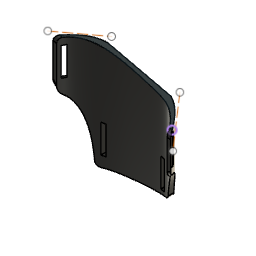
Back Hand Exo Bottom v4-flex material version v2 (Autodesk Fusion 360 design; units mm, degrees)
Autodesk Fusion 360 part; units mm, degrees
sketch "Base" plane through (0, 0, 0) normal (0, 0, 1) x (1, 0, 0)
  spline S0 degree 5 poles (14.4752, -0.0001) (14.6938, 0.8156) (15.231, 2.4269) (16.338, 4.7834) (18.4093, 7.7764) (22.0639, 11.0963) (26.9085, 13.7883) (33.3851, 15.6119) (41.8139, 16.4597) (51.3186, 16.5539) (60.7436, 16.1818) (68.8276, 15.6297) (74.9011, 14.9312) (78.8611, 13.937) (82.7401, 11.6359) (87.0744, 7.9841) (90.1424, 4.6022) (91.6876, 2.194) (92.2847, 0.711) (92.4752, 0) knots 0 0 0 0 0 0 0.066667 0.133333 0.2 0.266667 0.333333 0.4 0.466667 0.533333 0.6 0.666667 0.733333 0.8 0.866667 0.933333 1 1 1 1 1 1
  line L0 (12.4519, -7.5513) -> (16.4985, 7.551)
  line L1 (0, 0) -> (130, 0) construction
  line L2 (90.742, 6.4684) -> (94.2084, -6.4684)
  line L3 (72.0197, 16) -> (83.6365, 12)
  line L4 (20.0406, 11.0956) -> (36.9098, 16.9041)
  line L5 (28.4752, 32.4834) -> (28.4752, -47.2676) construction
  line L6 (79.3904, 33.3073) -> (79.3904, -47.7619) construction
  line L7 (14.4752, -0.0001) -> (11.9752, 0)
  line L8 (94.9752, 0) -> (92.4752, 0)
  line L9 (30.9752, 19.2841) -> (75.9752, 19.2841)
  line L10 (53.4752, 19.2841) -> (53.4752, -22.3142) construction
  spline S1 degree 5 poles (11.9752, 0) (12.2539, 0.5131) (12.8175, 1.532) (13.6807, 3.039) (14.8682, 5.0045) (16.4196, 7.3808) (18.0501, 9.6607) (19.7785, 11.8195) (21.6298, 13.823) (23.6348, 15.6281) (25.8277, 17.186) (27.7599, 18.1954) (29.322, 18.8009) (30.4155, 19.1347) (30.9752, 19.2841) knots 0 0 0 0 0 0 0.1 0.2 0.3 0.4 0.5 0.6 0.7 0.8 0.9 1 1 1 1 1 1
  spline S2 degree 5 poles (75.9752, 19.2841) (76.4009, 19.11) (77.2437, 18.7386) (78.4821, 18.1116) (80.0848, 17.1367) (82.0223, 15.6904) (83.9126, 14.0207) (85.7738, 12.1331) (87.6197, 10.0413) (89.4589, 7.7667) (91.2965, 5.3302) (92.7672, 3.2651) (93.871, 1.6557) (94.6071, 0.5563) (94.9752, 0) knots 0 0 0 0 0 0 0.1 0.2 0.3 0.4 0.5 0.6 0.7 0.8 0.9 1 1 1 1 1 1
  line L11 (27.5864, 18.3796) -> (34.364, 20.1885)
  line L12 (72.8438, 20.5644) -> (79.1066, 18.0038)
  point P0 (28.4752, 13.9999)
  point P1 (77.8281, 14)
  point P2 (20, 12)
  point P3 (84.8904, 13)
  dimension "d1" = 78
  dimension "d3" = 14
  dimension "d4" = 14
  dimension "d5" = 14
  dimension "d6" = 75
  dimension "d7" = 75
  dimension "d8" = 19
  dimension "d9" = 19
  dimension "d10" = 2.5
  dimension "d11" = 2.5
  dimension "d71" = 45
  dimension "d72" = 39
  dimension "d109" = 5.5
  constraint midpoint S0.start L0
  constraint coincident L1.start origin
  constraint horizontal L1
  constraint midpoint S0.end L2
  constraint midpoint P1 L3
  constraint midpoint P0 L4
  constraint coincident L1 L7.end
  constraint coincident L1 L8.start
  constraint perpendicular L1 L5
  constraint vertical L6
  constraint coincident P0 L5
  constraint coincident S0.end L1
  constraint perpendicular L5 L9
  constraint vertical L10
  constraint midpoint L9 L10.start
  constraint midpoint L9.start L11
  constraint midpoint L9.end L12
  measures "d1" distance of S0.start S0.end
  measures "d3" distance of S0.start P0
  measures "d4" distance of S0.start P0
  measures "d5" distance of P1 S0.end
  measures "d6" angle of L0 L1
  measures "d7" angle of L1 L2
  measures "d8" angle of L1 L3
  measures "d9" angle of L1 L4
  measures "d10" distance of S0.end L8.start
  measures "d11" distance of S0.start L7.end
  measures "d71" distance of L9.start L9.end
  measures "d72" distance of S0.start L10
  measures "d109" distance of L6 P3
extrude "Extrude1" add sketch "Base" along normal blind 80
ref_plane "WorkPlane1" through (0, 34, 0) normal (0, 1, 0) x (0, 0, 1)
ref_plane "WorkPlane2" through (0, -2, 0) normal (0, 1, 0) x (0, 0, 1)
sketch "Bottom cut" plane through (0, -2, 0) normal (0, 1, 0) x (1, 0, 0)
  line L0 (104.8084, -92.0022) -> (104.8084, 18.1008) construction
  line L1 (124.2592, 0) -> (-25.481, 0) construction
  line L2 (7.8084, -95.0569) -> (7.8084, 27.3148) construction
  line L3 (10.7244, 0) -> (10.7244, -80) construction
  line L4 (100.7244, 0) -> (100.7244, -80) construction
  line L5 (-40, -55.0042) -> (-40, 40)
  line L6 (-40, 40) -> (120.0224, 40)
  line L7 (120.0224, 40) -> (120.0224, -37.9442)
  line L8 (120.0224, -37.9442) -> (104.8084, -36.9507)
  spline S0 degree 5 poles (4.5707, -55.0042) (5.4547, -54.2774) (7.185, -52.7903) (9.6672, -50.4587) (12.7463, -47.1447) (16.1864, -42.6382) (19.185, -37.7387) (21.7128, -32.42) (23.7655, -26.6781) (25.3732, -20.5401) (26.5747, -14.0405) (27.2401, -8.5774) (27.5837, -4.3416) (27.7449, -1.4573) (27.8084, 0) knots 0 0 0 0 0 0 0.1 0.2 0.3 0.4 0.5 0.6 0.7 0.8 0.9 1 1 1 1 1 1
  spline S1 degree 5 poles (104.8084, -36.9507) (103.912, -36.7934) (102.1545, -36.4375) (99.6247, -35.7798) (96.4678, -34.651) (92.9056, -32.7929) (89.7589, -30.451) (87.057, -27.591) (84.8075, -24.2043) (82.9839, -20.3215) (81.5503, -15.9845) (80.6881, -12.1834) (80.191, -9.1584) (79.9251, -7.0655) (79.8084, -6) knots 0 0 0 0 0 0 0.1 0.2 0.3 0.4 0.5 0.6 0.7 0.8 0.9 1 1 1 1 1 1
  line L9 (79.8084, -6) -> (27.8084, 0)
  line L10 (4.5707, -55.0042) -> (-40, -55.0042)
  point P0 (20.8084, -34.1255)
  point P1 (87.8084, -28.2303)
  dimension "d50" = 20
  dimension "d51" = 13
  dimension "d52" = 17
  dimension "d53" = 25
  dimension "d54" = 97
  dimension "d55" = 6
  constraint vertical L0
  constraint perpendicular L0 L1
  constraint perpendicular L1 L2
  constraint coincident origin L1
  constraint coincident L0 L8.end
  constraint perpendicular L5 L6
  constraint perpendicular L6 L7
  constraint vertical L5
  constraint perpendicular L5 L10
  constraint coincident L1 S0.end
  constraint midpoint L0 L8.end
  measures "d50" distance of L2 S0.end
  measures "d51" distance of L2 P0
  measures "d52" distance of L0 P1
  measures "d53" distance of L0 S1.end
  measures "d54" distance of L0 L2
  measures "d55" distance of L1 S1.end
sketch "Top cut" plane through (0, -2, 0) normal (0, 1, 0) x (1, 0, 0)
  line L0 (101.7244, -58) -> (2.8084, -81)
  line L1 (2.8084, -81) -> (2.8084, -105)
  line L2 (2.8084, -105) -> (101.7244, -105)
  line L3 (101.7244, -105) -> (101.7244, -58)
  line L4 (100.7244, -80) -> (10.7244, -80)
  line L5 (7.8084, -95.0569) -> (7.8084, 27.3148)
  line L6 (100.7244, 0) -> (100.7244, -80)
  dimension "d41" = 22
  dimension "d42" = 1
  dimension "d43" = 5
  dimension "d44" = 25
  dimension "d49" = 1
  constraint vertical L1
  constraint perpendicular L1 L2
  constraint perpendicular L2 L3
  measures "d41" distance of L0.start L4
  measures "d42" distance of L0.end L4
  measures "d43" distance of L1 L5
  measures "d44" distance of L2 L4
  measures "d49" distance of L3 L6
extrude "Extrude4" cut sketch "Bottom cut" along normal blind 40
extrude "Extrude5" cut sketch "Top cut" along normal blind 55
fillet "Fillet5" radius 3 6 edges at (27.8084, 15.9515, 0) (79.8084, 15.2105, 6) (13.2252, -0.0001, 78.5779) (93.7252, 0, 59.86) (13.2515, -0.0001, 46.3199) (93.7045, 0, 33.0925)
sketch "Strap holes1-2" plane through (0, 19.2841, 0) normal (0, 1, 0) x (-1, 0, 0)
  line L0 (-30.9752, 0.3654) -> (-30.9752, 74.4507)
  line L1 (-30.9752, 74.4507) -> (-75.9752, 63.9872)
  line L2 (-75.9752, 63.9872) -> (-75.9752, 5.5577)
  line L3 (-75.9752, 5.5577) -> (-30.9752, 0.3654)
  line L4 (-75.9752, 28) -> (-72.9752, 28)
  line L5 (-72.9752, 28) -> (-72.9752, 8)
  line L6 (-72.9752, 8) -> (-75.9752, 8)
  line L7 (-75.9752, 8) -> (-75.9752, 28)
  line L8 (-33.9752, 28) -> (-30.9752, 28)
  line L9 (-30.9752, 28) -> (-30.9752, 8)
  line L10 (-30.9752, 8) -> (-33.9752, 8)
  line L11 (-33.9752, 8) -> (-33.9752, 28)
  dimension "d86" = 20
  dimension "d87" = 8
  dimension "d88" = 8
  dimension "d89" = 3
  constraint horizontal L4
  constraint vertical L5
  constraint horizontal L6
  constraint vertical L7
  constraint horizontal L8
  constraint vertical L9
  constraint horizontal L10
  constraint vertical L11
  constraint equal L5 L9
  constraint equal L6 L10
  constraint collinear L2 L7
  constraint collinear L0 L9
  measures "d86" distance of L8.end L9.end
  measures "d87" distance of origin L6
  measures "d88" distance of origin L10
  measures "d89" distance of L8.start L8.end
extrude "Extrude9" cut sketch "Strap holes1-2" against normal blind 12 contours L0 L8 L9 L10 L11 | L2 L4 L5 L6 L7
sketch "Construction lines" plane through (18.0122, 0, 77.4648) normal (0.226479, 0, 0.974016) x (0, 1, 0)
  line L0 (3, -74.9955) -> (3, -76.9235)
  spline S0 degree 3 poles (19.2841, -59.5093) (18.5382, -61.3823) (17.5569, -63.1027) (15.0981, -66.4885) (13.6124, -68.1026) (9.3648, -72.1628) (6.1133, -74.6914) (3, -76.9235) knots -2.622013 -2.622013 -2.622013 -2.622013 -2.044383 -2.044383 -1.421419 -1.421419 -0.351491 -0.351491 -0.351491 -0.351491
  line L1 (19.2841, -59.5093) -> (19.2841, -13.3088)
  spline S1 degree 3 poles (2.9999, 4.4524) (5.1721, 3.1335) (7.3375, 1.6927) (12.1853, -2.017) (14.2699, -4.0868) (17.4499, -8.3262) (18.5944, -10.6561) (19.2841, -13.3088) knots -2.116349 -2.116349 -2.116349 -2.116349 -1.596237 -1.596237 -0.822275 -0.822275 0 0 0 0
  line L2 (2.9999, 4.4524) -> (2.9998, 2.5008)
  spline S2 degree 3 poles (3, -74.9955) (3.0917, -74.9346) (3.1848, -74.8715) (4.4933, -73.9667) (5.6856, -72.9258) (8.6937, -69.9863) (10.9302, -67.3764) (13.9428, -62.2377) (14.6004, -59.9316) (15.9248, -50.1325) (16.8031, -35.3469) (16.1369, -21.9872) (15.8285, -18.5893) (14.5153, -11.8314) (13.4247, -8.5439) (10.1138, -3.0136) (8.204, -0.9569) (5.1534, 1.3241) (4.1036, 1.9675) (2.9998, 2.5008) knots -9.571922 -9.571922 -9.571922 -9.571922 -9.507415 -9.507415 -8.679656 -8.679656 -7.14863 -7.14863 -5.628617 -5.628617 -3.129046 -3.129046 -2.35518 -2.35518 -1.469689 -1.469689 -0.691384 -0.691384 -0.321973 -0.321973 -0.321973 -0.321973
  line L3 (0, 10) -> (24.0161, -11.5563) construction
  line L4 (25, -60) -> (-7.1736, -87.8504) construction
ref_plane "WorkPlane3" through (18.7701, 12.0081, 77.2886) normal (0.752855, -0.658187, 0) x (0.650612, 0.74419, -0.151281)
ref_plane "WorkPlane4" through (90.0165, 8.9132, 60.7223) normal (-0.764523, -0.644597, 0) x (0.637476, -0.756077, -0.148226)
sketch "Strap hole3" plane through (18.7701, 12.0081, 77.2886) normal (0.752855, -0.658187, 0) x (0.650612, 0.74419, -0.151281)
  line L0 (-16.1358, 0) -> (16.1358, 0)
  line L1 (-13.8484, 1.1658) -> (-7.7972, -38.3738) construction
  line L2 (-9.5712, -26.7821) -> (-13.1302, -3.527) construction
  line L3 (-8.7786, -5.5204) -> (-5.753, -25.2902)
  line L4 (-5.753, -25.2902) -> (-2.7875, -24.8363)
  line L5 (-2.7875, -24.8363) -> (-5.8131, -5.0665)
  line L6 (-5.8131, -5.0665) -> (-8.7786, -5.5204)
  dimension "d97" = 40
  dimension "d98" = 20
  dimension "d99" = 3
  dimension "d108" = 4
  constraint parallel L1 L2
  constraint collinear L1 L2
  constraint parallel L1 L3
  constraint perpendicular L3 L4
  constraint perpendicular L3 L6
  constraint parallel L3 L5
  measures "d97" distance of L1.start L1.end
  measures "d98" distance of L3.start L3.end
  measures "d99" distance of L3.end L4.end
  measures "d108" distance of L1 L3
extrude "Extrude10" cut sketch "Strap hole3" along normal blind 15
sketch "Strap hole4" plane through (90.0165, 8.9132, 60.7223) normal (-0.764523, -0.644597, 0) x (0.637476, -0.756077, -0.148226)
  line L0 (9.0547, 7.1245) -> (15.1012, -33.2171) construction
  line L1 (13.3992, -21.8617) -> (10.5276, -2.7024) construction
  line L2 (6.2026, -3.1012) -> (9.0051, -22.9039)
  line L3 (6.2026, -3.1012) -> (3.2322, -3.5216)
  line L4 (3.2322, -3.5216) -> (6.0347, -23.3243)
  line L5 (6.0347, -23.3243) -> (9.0051, -22.9039)
  dimension "d102" = 20
  dimension "d103" = 4.5
  dimension "d105" = 3
  constraint collinear L0 L1
  constraint perpendicular L2 L3
  constraint perpendicular L3 L4
  constraint perpendicular L4 L5
  measures "d102" distance of L2.start L2.end
  measures "d103" distance of L0 L2.end
  measures "d105" distance of L2.start L3.end
extrude "Extrude11" cut sketch "Strap hole4" along normal blind 20
sketch "Sketch15" plane through (18.7701, 12.0081, 77.2886) normal (0.752855, -0.658187, 0) x (0.650612, 0.74419, -0.151281)
equation "d72 = ( 78 / 2 ) * 1 mm"
